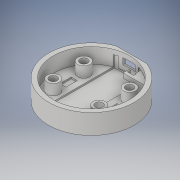
# Autodesk Inventor part: Base
Saved by Autodesk Inventor 2019 (Build 230136000, 136)
## iProperties
Created: 2019-10-05
Part Number: Base
Material: Generic
Document SubType Name: Modeling
Designer: Josiah
Density: 1 g/cm^3
Appearance: Default
Author: Josiah
Autodesk Inventor part; units mm, degrees
ref_plane "YZ Plane" through (0, 0, 0) normal (1, 0, 0) x (0, 1, 0)
ref_plane "XZ Plane" through (0, 0, 0) normal (0, 1, 0) x (-1, 0, 0)
ref_plane "XY Plane" through (0, 0, 0) normal (0, 0, 1) x (1, 0, 0)
sketch "Sketch1" plane through (0, 0, 0) normal (0, 1, 0) x (-1, 0, 0)
  line L0 (8.5, 21.5) -> (-8.5, 21.5) construction
  line L1 (-8.5, 21.5) -> (-8.5, -21.5) construction
  line L2 (8.5, -21.5) -> (8.5, 21.5) construction
  line L3 (-8.5, 21.5) -> (8.5, -21.5) construction
  line L4 (-8.5, -21.5) -> (8.5, 21.5) construction
  line L5 (-3.5, -21.5) -> (-3.5, -23.5) construction
  line L6 (-3.5, -23.5) -> (3.5, -23.5) construction
  line L7 (3.5, -23.5) -> (3.5, -21.5) construction
  line L8 (-8.5, -21.5) -> (-3.5, -21.5) construction
  line L9 (3.5, -21.5) -> (8.5, -21.5) construction
  arc A0 (9.5253, -23.1034) -> (-9.5253, -23.1034) centre (0, 0) ccw
  line L10 (9.5253, -23.1034) -> (-9.5253, -23.1034)
  line L11 (-10.102, -26.1034) -> (10.102, -26.1034)
  arc A1 (10.102, -26.1034) -> (-10.102, -26.1034) centre (0, 0) ccw
  dimension "d0" = 43
  dimension "d1" = 17
  dimension "d2" = 7
  dimension "d3" = 2
  dimension "d4" = 3
  dimension "d13" = 20.204
  constraints: 24 end point, 4 parallel, 4 point on circle, 2 centre point, 1 coincident, 1 horizontal, 1 perpendicular, 1 other
  measures "d0" distance of L2.start L0.start
  measures "d1" distance of L1.end L2.start
  measures "d2" distance of L5.end L6.end
  measures "d3" distance of L5.start L5.end
  measures "d4" radial gap between concentric circles of A0 A1
  measures "d13" distance of L11.start L11.end
extrude "BASE PLATE" add sketch "Sketch1" along normal blind 3 contours L10 A0 | A1 L11
sketch "Sketch3" plane through (0, 3, 0) normal (0, 1, 0) x (1, 0, 0)
  line L0 (10.102, 26.1034) -> (-10.102, 26.1034) projected
  arc A0 (-10.102, 26.1034) -> (10.102, 26.1034) centre (0, 0) ccw
  arc A1 (-10.102, 26.1034) -> (10.102, 26.1034) centre (0, 0) ccw projected
  line L1 (-10.102, 26.1034) -> (10.102, 26.1034)
  circle A2 centre (0, 0) radius 24.99
  dimension "d58" = 3
  constraints: 4 coincident, 3 end point, 2 centre point, 2 point on circle, 1 collinear, 4 other
  measures "d58" radial gap between concentric circles of A0 A2
extrude "WALLS" add sketch "Sketch3" along normal blind 10
sketch "Sketch6" plane through (0, 3, 0) normal (0, 1, 0) x (1, 0, 0)
  line L0 (-8.5, 21.5) -> (8.5, 21.5) construction
  line L1 (8.5, 21.5) -> (8.5, -21.5) construction
  line L2 (8.5, -21.5) -> (-8.5, -21.5) construction
  line L3 (-8.5, -21.5) -> (-8.5, 21.5) construction
  line L4 (-8.5, -21.5) -> (8.5, 21.5) construction
  line L5 (-8.5, 21.5) -> (8.5, -21.5) construction
  line L6 (0, 0) -> (-15, 0) construction
  line L7 (-15, 0) -> (-15, 10) construction
  line L8 (-15, 10) -> (0, 10) construction
  line L9 (0, 10) -> (0, 0) construction
  circle A0 centre (-15, 10) radius 4
  circle A1 centre (-15, 10) radius 2.5
  circle A2 centre (-15, -10) radius 4
  circle A3 centre (-15, -10) radius 2.5
  circle A4 centre (15, 10) radius 4
  circle A5 centre (15, 10) radius 2.5
  circle A6 centre (15, -10) radius 2.5
  circle A7 centre (15, -10) radius 4
  dimension "d18" = 43
  dimension "d19" = 17
  dimension "d20" = 15
  dimension "d21" = 10
  dimension "d22" = 8
  dimension "d23" = 5
  constraints: 20 end point, 8 centre point, 6 symmetric about line, 5 coincident, 4 parallel, 2 horizontal, 2 perpendicular, 6 other
  measures "d18" distance of L0.end L1.end
  measures "d19" distance of L0.start L0.end
  measures "d20" distance of L7.end L8.end
  measures "d21" distance of L6.end L7.end
  measures "d22" diameter of A0
  measures "d23" diameter of A1
extrude "BUTTON POSTS" add sketch "Sketch6" along normal blind 7
sketch "Sketch7" plane through (0, 3, 0) normal (0, 1, 0) x (1, 0, 0)
  line L0 (-9, 24.1034) -> (9, 24.1034)
  line L1 (9, 24.1034) -> (9, -19.0966)
  line L2 (9, -19.0966) -> (-9, -19.0966)
  line L3 (-9, -19.0966) -> (-9, 24.1034)
  line L4 (-17, 3.75) -> (-13, 3.75)
  line L5 (-13, 3.75) -> (-13, -3.75)
  line L6 (-13, -3.75) -> (-17, -3.75)
  line L7 (-17, -3.75) -> (-17, 3.75)
  line L8 (-24.99, 0) -> (24.99, 0) construction
  line L9 (0, 23.1034) -> (0, -24.99) construction
  line L10 (17, 3.75) -> (13, 3.75)
  line L11 (13, 3.75) -> (13, -3.75)
  line L12 (13, -3.75) -> (17, -3.75)
  line L13 (17, -3.75) -> (17, 3.75)
  line L14 (-9.5253, 24.1034) -> (9.5253, 24.1034) projected
  line L15 (10.102, 26.1034) -> (-10.102, 26.1034) projected
  dimension "d26" = 43.2
  dimension "d27" = 18
  dimension "d28" = 7.5
  dimension "d29" = 4
  dimension "d30" = 3.75
  dimension "d63" = 2
  dimension "d65" = 9
  dimension "d77" = 13
  constraints: 28 end point, 4 horizontal, 4 parallel, 4 symmetric about line, 2 perpendicular, 1 vertical
  measures "d26" distance of L2.end L0.start
  measures "d27" distance of L0.start L0.end
  measures "d28" distance of L4.end L5.end
  measures "d29" distance of L4.start L4.end
  measures "d30" distance between parallel lines of L4 L8
  measures "d63" distance between parallel lines of L0 L15
  measures "d65" distance between parallel lines of L9 L3
  measures "d77" distance between parallel lines of L5 L9
extrude "INDENTATION FOR LINEUP" cut sketch "Sketch7" against normal blind 1
sketch "Sketch9" plane through (0, 2, 0) normal (0, 1, 0) x (1, 0, 0)
  line L0 (-9, 24.1034) -> (9, 24.1034) projected
  line L1 (-9, -19.0966) -> (9, -19.0966)
  line L2 (9, -19.0966) -> (9, 24.1034)
  line L3 (9, 24.1034) -> (-9, 24.1034)
  line L4 (-9, 24.1034) -> (-9, -19.0966)
  point P0 (0, 0)
  constraints: 8 end point, 2 parallel, 1 horizontal, 1 perpendicular
extrude "FLAT SURFACE FOR ARDUINO" cut sketch "Sketch9" along normal blind 8
sketch "Sketch11" plane through (10.102, 0, -26.1034) normal (0, 0, -1) x (-1, 0, 0)
  line L0 (19.102, 2) -> (1.102, 2) construction
  line L1 (0, 0) -> (0, 13) construction
  line L2 (20.204, 0) -> (20.204, 13) construction
  line L3 (6.1, 10) -> (14.1, 10)
  line L4 (14.1, 10) -> (14.1, 6)
  line L5 (14.1, 6) -> (6.1, 6)
  line L6 (6.1, 6) -> (6.1, 10)
  line L7 (0, 0) -> (20.204, 0) construction
  circle A0 centre (2.5, 9.5) radius 1
  point P0 (10.102, 0)
  dimension "d69" = 4
  dimension "d70" = 4
  dimension "d71" = 6.1
  dimension "d72" = 2
  dimension "d74" = 2.5
  dimension "d78" = 7.5
  dimension "d89" = 8
  constraints: 8 end point, 2 parallel, 1 centre point, 1 horizontal, 1 perpendicular
  measures "d69" distance of L3.end L4.end
  measures "d70" distance between parallel lines of L5 L0
  measures "d71" distance between parallel lines of L1 L6
  measures "d72" diameter of A0
  measures "d74" distance from line of L1 A0.centre
  measures "d78" distance from line of A0.centre L0
  measures "d89" distance of L3.start L3.end
extrude "I/O HOLES" cut sketch "Sketch11" against normal blind 10
sketch "Sketch12" plane through (0, 3, 0) normal (0, 1, 0) x (1, 0, 0)
  line L0 (19.1097, 16.1034) -> (9, 16.1034)
  line L1 (9, 16.1034) -> (9, 23.3131)
  line L2 (-9, 24.1034) -> (9, 24.1034) construction
  line L3 (-9, -19.0966) -> (-9, 24.1034) construction
  line L4 (9, -19.0966) -> (-9, -19.0966) construction
  line L5 (9, 24.1034) -> (9, -19.0966) construction
  line L6 (10.102, 26.1034) -> (-10.102, 26.1034) projected
  circle A0 centre (0, 0) radius 24.99 construction
  arc A1 (-9, 23.3131) -> (9, 23.3131) centre (0, 0) ccw projected
  arc A2 (19.1097, 16.1034) -> (9, 23.3131) centre (0, 0) ccw
  line L7 (9, 23.3131) -> (9, -19.0966) projected
  point P0 (13, 21.3424)
  dimension "d88" = 10
  constraints: 4 end point, 4 point on circle, 1 centre point, 1 coincident, 1 collinear, 1 concentric, 1 horizontal, 1 point on line, 1 vertical, 4 other
  measures "d88" distance between parallel lines of L6 L0
extrude "Extrusion11" add sketch "Sketch12" along normal blind 7
sketch "Sketch15" plane through (0, 10, 0) normal (0, 1, 0) x (1, 0, 0)
  line L0 (9, 23.3131) -> (9, 16.1034) construction
  line L1 (9, 16.1034) -> (19.1097, 16.1034) construction
  arc A0 (19.1097, 16.1034) -> (9, 23.3131) centre (0, 0) ccw construction
  line L2 (6.602, 26.1034) -> (8.602, 26.1034) construction
  line L3 (8.468, 24.1034) -> (6.736, 24.1034) construction
  line L4 (7.602, 26.1034) -> (7.602, 18.0057) construction
  line L5 (5.602, 19.8034) -> (9.602, 19.8034) construction
  line L6 (9.602, 19.8034) -> (9.602, 18.1034) construction
  line L7 (9.602, 18.1034) -> (5.602, 18.1034) construction
  line L8 (5.602, 18.1034) -> (5.602, 19.8034) construction
  line L9 (9, 19.8034) -> (9.602, 19.8034)
  line L10 (9.602, 19.8034) -> (9.602, 18.1034)
  line L11 (9.602, 18.1034) -> (9, 18.1034)
  line L12 (9, 18.1034) -> (9, 19.8034)
  line L13 (8.468, 23.5115) -> (8.468, 24.1034) projected
  line L14 (6.736, 24.1034) -> (6.736, 24.065) projected
  point P0 (8.602, 24.1034)
  point P1 (6.602, 24.1034)
  point P2 (9, 19.7083)
  dimension "d90" = 4
  dimension "d91" = 2
  dimension "d92" = 1.7
  dimension "d93" = 2
  constraints: 18 end point, 4 parallel, 2 horizontal, 2 midpoint, 2 perpendicular, 2 point on line, 1 vertical, 1 other
  measures "d90" distance of L5.start L5.end
  measures "d91" distance between parallel lines of L4 L8
  measures "d92" distance of L7.end L5.start
  measures "d93" distance between parallel lines of L7 L1
extrude "Extrusion12" cut sketch "Sketch15" against normal blind 2.3
sketch "Sketch16" plane through (9, 2, -24.1034) normal (-1, 0, 0) x (0, 0, 1)
  line L0 (0, 8) -> (0, 6.5) construction
  line L1 (6, 8) -> (8, 8) construction
  line L2 (6, 8) -> (6, 5.7) construction
  line L3 (6, 5.7) -> (4.3, 5.7) construction
  line L4 (4.3, 5.7) -> (4.3, 8) construction
  line L5 (0.7903, 8) -> (4.3, 8) construction
  line L6 (8, 1) -> (8, 8) construction
  line L7 (6, 8) -> (8, 8) construction
  line L8 (14.8538, 7.25) -> (0, 7.25) construction
  line L9 (0, 0) -> (0, 8) construction
  line L10 (6, 8) -> (8, 8)
  line L11 (8, 8) -> (8, 5)
  line L12 (8, 5) -> (6, 5)
  line L13 (6, 5) -> (6, 8)
  point P0 (24.1034, -2)
  dimension "d96" = 3
  dimension "d97" = 2
  constraints: 10 end point, 2 horizontal, 2 parallel, 1 midpoint, 1 perpendicular, 1 point on line
  measures "d96" distance of L1.end L11.end
  measures "d97" distance of L1.end L10.start
extrude "Extrusion13" add sketch "Sketch16" along normal blind 4.398
sketch "Sketch17" plane through (9.602, 7.7, -18.1034) normal (0, 0, -1) x (-1, 0, 0)
  line L0 (5, -0.7) -> (4.2, -0.7)
  line L1 (4.2, -0.7) -> (4.2, 2.3)
  line L2 (4.2, 2.3) -> (5, 2.3)
  line L3 (5, 2.3) -> (5, -0.7)
  point P0 (9.602, -7.7)
  dimension "d100" = 3
  dimension "d101" = 0.8
  constraints: 8 end point, 2 parallel, 1 coincident, 1 horizontal, 1 perpendicular
  measures "d100" distance of L0.end L1.end
  measures "d101" distance of L1.end L2.end
extrude "Extrusion14" add sketch "Sketch17" along normal blind 2
equation "\"d30\" = 0.5 * d28"
equation "\"d65\" = 0.5 * d27"
equation "\"d91\" = 0.5 * d90"
body "Solid1"
